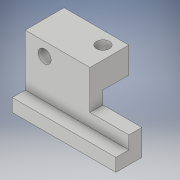
# Autodesk Inventor part: Part3
Saved by Autodesk Inventor 2017 (Build 210142000, 142)
## iProperties
Created: 2016-11-01
Part Number: Part3
Material: Generic
Document SubType Name: Modeling
Designer: s411888
Density: 1 g/cm^3
Appearance: Default
Author: s411888
Autodesk Inventor part; units mm, degrees
ref_plane "YZ Plane" through (0, 0, 0) normal (1, 0, 0) x (0, 1, 0)
ref_plane "XZ Plane" through (0, 0, 0) normal (0, 1, 0) x (-1, 0, 0)
ref_plane "XY Plane" through (0, 0, 0) normal (0, 0, 1) x (1, 0, 0)
sketch "Sketch1" plane through (0, 0, 0) normal (1, 0, 0) x (0, 1, 0)
  line L0 (-3.4784, 6.7709) -> (-9.8284, 6.7709)
  line L1 (-9.8284, 6.7709) -> (-9.8284, -5.9291)
  line L2 (-9.8284, -5.9291) -> (-3.4784, -5.9291)
  line L3 (-3.4784, -5.9291) -> (-3.4784, 6.7709)
  line L4 (-9.8092, -5.9291) -> (2.8908, -5.9291)
  line L5 (2.8908, -5.9291) -> (2.8908, 0.4209)
  line L6 (2.8908, 0.4209) -> (-9.8092, 0.4209)
  line L7 (-9.8092, 0.4209) -> (-9.8092, -5.9291)
  line L8 (2.8908, 0.4209) -> (21.9408, 0.4209)
  line L9 (21.9408, 0.4209) -> (21.9408, -5.9291)
  line L10 (21.9408, -5.9291) -> (2.8908, -5.9291)
  line L11 (2.8908, -5.9291) -> (2.8908, 0.4209)
  line L12 (21.9408, 0.4209) -> (9.2408, 0.4209)
  line L13 (9.2408, 0.4209) -> (9.2408, -18.6291)
  line L14 (9.2408, -18.6291) -> (21.9408, -18.6291)
  line L15 (21.9408, -18.6291) -> (21.9408, 0.4209)
  point P0 (0, 0)
  dimension "d0" = 6.35
  dimension "d1" = 12.7
  dimension "d2" = 12.7
  dimension "d3" = 6.35
  dimension "d4" = 19.05
  dimension "d5" = 6.35
  dimension "d6" = 12.7
  dimension "d7" = 19.05
  constraints: 32 end point, 8 parallel, 4 horizontal, 4 perpendicular, 1 point on line
  measures "d0" distance of L2.end L1.end
  measures "d1" distance of L1.end L0.end
  measures "d2" distance of L6.end L5.end
  measures "d3" distance of L5.end L4.end
  measures "d4" distance of L9.end L10.end
  measures "d5" distance of L8.end L9.end
  measures "d6" distance of L14.end L13.end
  measures "d7" distance of L13.end L12.end
extrude "Extrusion1" add sketch "Sketch1" along normal blind 50.8 contours L3 L6 L7 L2 L1 L0 | L3 L2 L7 L6
extrude "Extrusion2" add sketch "Sketch1" along normal blind 31.75 contours L8 L13 L10 L5 | L8 L9 L10 L13
extrude "Extrusion3" cut sketch "Sketch1" along normal blind 50.8 contours L6 L5 L4 L3 | L3 L2 L7 L6
extrude "Extrusion4" add sketch "Sketch1" along normal blind 50.8 contours L6 L5 L4 L3 | L3 L2 L7 L6
extrude "Extrusion5" cut sketch "Sketch1" along normal blind 31.75 contours L8 L9 L10 L13 | L10 L15 L14 L13
extrude "Extrusion6" add sketch "Sketch1" along normal blind 31.75 contours L8 L9 L10 L13 | L10 L15 L14 L13
sketch "Sketch2" plane through (0, 21.9408, 0.4209) normal (0, 1, 0) x (1, 0, 0)
  line L0 (31.75, 12.7) -> (31.75, 19.05)
  circle A0 centre (25.4, 12.7) radius 3.175
  point P0 (0, 0.4209)
  dimension "d22" = 6.35
  constraints: 2 end point, 1 centre point
  measures "d22" diameter of A0
extrude "Extrusion7" cut sketch "Sketch2" against normal blind 12.7
sketch "Sketch3" plane through (0, -3.4784, 0.4209) normal (0, 0, 1) x (1, 0, 0)
  line L0 (0, 12.7192) -> (0, 25.4192) projected
  line L1 (0, 25.4192) -> (6.35, 25.4192)
  line L2 (0, 19.0692) -> (0, 25.4192)
  line L3 (6.35, 25.4192) -> (9.525, 25.4192)
  line L4 (9.525, 19.0692) -> (6.35, 19.0692)
  circle A0 centre (9.525, 19.0692) radius 3.175
  point P0 (0, 3.4784)
  dimension "d27" = 3.175
  dimension "d28" = 6.35
  dimension "d29" = 6.35
  constraints: 8 end point, 2 horizontal, 1 centre point, 1 coincident, 1 parallel
  measures "d27" distance of L4.start L4.end
  measures "d28" distance of L3.end L4.start
  measures "d29" diameter of A0
extrude "Extrusion8" cut sketch "Sketch3" against normal blind 25.4
body "Solid1"
